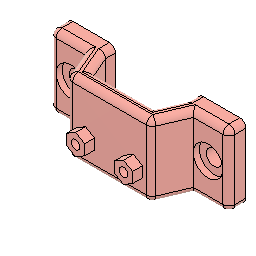
Z Leadscrew Nut to Bed Mount v7 (Autodesk Fusion 360 design; units mm, degrees)
Autodesk Fusion 360 part; units mm, degrees
sketch "Sketch1" plane through (0, 0, 0) normal (0, 0, 1) x (1, 0, 0) in component "Leadscrew Nut Mount V1"
  line L0 (0, 0) -> (0, 30)
  line L1 (0, 0) -> (73.8, 0)
  line L2 (73.8, 0) -> (73.8, 30)
  line L3 (73.8, 30) -> (0, 30)
  line L4 (36.9, 0) -> (36.9, 10) construction
  line L5 (36.9, 10) -> (27, 10) construction
  line L6 (36.9, 10) -> (46.8, 10) construction
  circle A0 centre (27, 10) radius 2.5
  circle A1 centre (46.8, 10) radius 2.5
  line L7 (29.9, 11.6743) -> (27, 13.3486)
  line L8 (27, 13.3486) -> (24.1, 11.6743)
  line L9 (24.1, 11.6743) -> (24.1, 8.3257)
  line L10 (24.1, 8.3257) -> (27, 6.6514)
  line L11 (27, 6.6514) -> (29.9, 8.3257)
  line L12 (29.9, 8.3257) -> (29.9, 11.6743)
  line L13 (43.9, 8.3257) -> (46.8, 6.6514)
  line L14 (46.8, 6.6514) -> (49.7, 8.3257)
  line L15 (49.7, 8.3257) -> (49.7, 11.6743)
  line L16 (49.7, 11.6743) -> (46.8, 13.3486)
  line L17 (46.8, 13.3486) -> (43.9, 11.6743)
  line L18 (43.9, 11.6743) -> (43.9, 8.3257)
  line L19 (0, 0) -> (20, 0)
  line L20 (20, 0) -> (20, 30)
  circle A2 centre (8.6, 15) radius 3.2
  circle A3 centre (8.6, 15) radius 6.1
  circle A4 centre (65.2, 15) radius 6.1
  circle A5 centre (65.2, 15) radius 3.2
  line L21 (53.8, 0) -> (53.8, 30)
  line L22 (0, 15) -> (8.6, 15) construction
  dimension "d1" = 10
  dimension "d2" = 5
  dimension "d3" = 5
  dimension "d4" = 9.9
  dimension "d5" = 2.9
  dimension "d6" = 2.9
  dimension "d21" = 73.8
  dimension "d22" = 6.4
  dimension "d23" = 12.2
  dimension "d24" = 30
  dimension "d25" = 33.8
  dimension "d26" = 8.6
  measures "d1" distance of L0.start
  measures "d2" diameter of A1
  measures "d3" diameter of A0
  measures "d5" distance of L18
  measures "d6" distance of L12
  measures "d22" diameter of A2
  measures "d23" diameter of A3
  measures "d25" distance of L20 L21
extrude "Extrude1" add sketch "Sketch1" along normal blind 7 contours L0 L1 L3 L19 L20 | L1 L2 L3 L21 | A3 | A4 makes body 1 at (64.187, 3.9363, 0) makes body 2 at (9.613, 3.9363, 0) in component "Leadscrew Nut Mount V1"
extrude "Extrude2" cut sketch "Sketch1" along normal through all from surface at 4.5 contours A3 | A4 bodies 1 2 in component "Leadscrew Nut Mount V1"
extrude "Extrude3" add sketch "Sketch1" along normal blind 2.75 from surface at 25.4 separate body contours L1 L3 L20 L21 makes body 3 in component "Leadscrew Nut Mount V1"
extrude "Extrude4" add sketch "Sketch1" along normal blind 3 from surface at 28.15 contours L1 L3 L20 L21 | L7 L8 L9 L10 L11 L12 | L13 L14 L15 L16 L17 L18 bodies 3 in component "Leadscrew Nut Mount V1"
sketch "Sketch2" plane through (0, 0, 0) normal (0, -1, 0) x (1, 0, 0) in component "Leadscrew Nut Mount V1"
  line L0 (20, 25.4) -> (53.8, 25.4)
  line L1 (53.8, 25.4) -> (53.8, 31.15)
  line L2 (53.8, 31.15) -> (20, 31.15)
  line L3 (20, 31.15) -> (20, 25.4)
  line L4 (59.1, 7) -> (71.3, 7)
  line L5 (53.8, 25.4) -> (53.8, 31.15)
  line L6 (53.8, 31.15) -> (59.1, 7)
  line L7 (53.8, 25.4) -> (48.2257, 25.4)
  line L8 (53.8, 0) -> (53.8, 7)
  line L9 (49.7, 25.4) -> (53.8, 6.7179)
  line L10 (59.1, 7) -> (53.8, 7)
  line L11 (53.8, 25.4) -> (20, 25.4)
  line L12 (20, 31.15) -> (53.8, 31.15)
  line L13 (36.9, 31.15) -> (36.9, 25.4)
  line L14 (24.1, 25.4) -> (20, 6.7179)
  line L15 (20, 31.15) -> (14.7, 7)
  line L16 (20, 25.4) -> (24.1, 25.4)
  line L17 (20, 25.4) -> (20, 31.15)
  line L18 (14.7, 7) -> (20, 7)
  line L19 (20, 0) -> (20, 7)
extrude "Extrude5" add sketch "Sketch2" against normal up to surface (30 mm away) contours L0 L3 L11 L14 L15 L16 L17 L18 L19 | L0 L1 L5 L6 L7 L8 L9 L10 L11 bodies 3 1 2 in component "Leadscrew Nut Mount V1"
fillet "Fillet1" radius 2.5 28 edges at (36.9, 30, 31.15) (17.35, 30, 19.075) (36.9, 30, 25.4) (22.05, 30, 16.059) (51.75, 30, 16.059) (56.45, 30, 19.075) (56.45, 0, 19.075) (51.75, 0, 16.059) (22.05, 0, 16.059) (17.35, 0, 19.075) (36.9, 0, 31.15) (53.8, 15, 31.15) (20, 15, 31.15) (20, 30, 3.359) (0, 30, 3.5) (7.35, 30, 7) (0, 15, 7) (7.35, 0, 7) (53.8, 30, 3.359) (66.45, 30, 7) (73.8, 30, 3.5) (73.8, 15, 7) (73.8, 0, 3.5) (66.45, 0, 7) (53.8, 0, 3.359) (36.9, 0, 25.4) (20, 0, 3.359) (0, 0, 3.5) on bodies 3 in component "Leadscrew Nut Mount V1"
sketch "Sketch1 (2)" plane through (0, 0, 0) normal (0, 0, 1) x (1, 0, 0) in component "Leadscrew Nut Mount V1.1"
  line L0 (0, 0) -> (0, 30)
  line L1 (0, 0) -> (73.8, 0)
  line L2 (73.8, 0) -> (73.8, 30)
  line L3 (73.8, 30) -> (0, 30)
  line L4 (36.9, 0) -> (36.9, 10) construction
  line L5 (36.9, 10) -> (27, 10) construction
  line L6 (36.9, 10) -> (46.8, 10) construction
  circle A0 centre (27, 10) radius 1.8
  circle A1 centre (46.8, 10) radius 1.8
  line L7 (29.9, 11.6743) -> (27, 13.3486)
  line L8 (27, 13.3486) -> (24.1, 11.6743)
  line L9 (24.1, 11.6743) -> (24.1, 8.3257)
  line L10 (24.1, 8.3257) -> (27, 6.6514)
  line L11 (27, 6.6514) -> (29.9, 8.3257)
  line L12 (29.9, 8.3257) -> (29.9, 11.6743)
  line L13 (43.9, 8.3257) -> (46.8, 6.6514)
  line L14 (46.8, 6.6514) -> (49.7, 8.3257)
  line L15 (49.7, 8.3257) -> (49.7, 11.6743)
  line L16 (49.7, 11.6743) -> (46.8, 13.3486)
  line L17 (46.8, 13.3486) -> (43.9, 11.6743)
  line L18 (43.9, 11.6743) -> (43.9, 8.3257)
  line L19 (0, 0) -> (20, 0)
  line L20 (20, 0) -> (20, 30)
  circle A2 centre (8.6, 15) radius 3.2
  circle A3 centre (8.6, 15) radius 6.1
  circle A4 centre (65.2, 15) radius 6.1
  circle A5 centre (65.2, 15) radius 3.2
  line L21 (53.8, 0) -> (53.8, 30)
  line L22 (0, 15) -> (8.6, 15) construction
  dimension "d1_1" = 10
  dimension "d2_1" = 3.6
  dimension "d3_1" = 3.6
  dimension "d4_1" = 9.9
  dimension "d5_1" = 2.9
  dimension "d6_1" = 2.9
  dimension "d21_1" = 73.8
  dimension "d22_1" = 6.4
  dimension "d23_1" = 12.2
  dimension "d24_1" = 30
  dimension "d25_1" = 33.8
  dimension "d26_1" = 8.6
  measures "d1_1" distance of L0.start
  measures "d2_1" diameter of A1
  measures "d3_1" diameter of A0
  measures "d5_1" distance of L18
  measures "d6_1" distance of L12
  measures "d22_1" diameter of A2
  measures "d23_1" diameter of A3
  measures "d25_1" distance of L20 L21
extrude "Extrude1'" add sketch "Sketch1 (2)" along normal blind 7 separate body contours L0 L1 L3 L19 L20 | L1 L2 L3 L21 | A3 | A4 makes body 4 at (64.187, 3.9363, 0) makes body 5 at (9.613, 3.9363, 0) in component "Leadscrew Nut Mount V1.1"
extrude "Extrude2'" cut sketch "Sketch1 (2)" along normal through all from surface at 4.5 contours A3 | A4 bodies 4 5 in component "Leadscrew Nut Mount V1.1"
extrude "Extrude3'" add sketch "Sketch1 (2)" along normal blind 2.75 from surface at 13.65 separate body contours L1 L3 L20 L21 makes body 6 in component "Leadscrew Nut Mount V1.1"
extrude "Extrude4'" add sketch "Sketch1 (2)" along normal blind 3 from surface at 16.4 contours L1 L3 L20 L21 | L7 L8 L9 L10 L11 L12 | L13 L14 L15 L16 L17 L18 bodies 6 in component "Leadscrew Nut Mount V1.1"
sketch "Sketch2 (2)" plane through (0, 0, 0) normal (0, -1, 0) x (1, 0, 0) in component "Leadscrew Nut Mount V1.1"
  line L0 (20, 13.65) -> (53.8, 13.65)
  line L1 (53.8, 13.65) -> (53.8, 19.4)
  line L2 (53.8, 19.4) -> (20, 19.4)
  line L3 (20, 19.4) -> (20, 13.65)
  line L4 (59.1, 7) -> (71.3, 7)
  line L5 (53.8, 13.65) -> (53.8, 19.4)
  line L6 (53.8, 19.4) -> (59.1, 7)
  line L7 (53.8, 13.65) -> (48.2257, 13.65)
  line L8 (53.8, 0) -> (53.8, 7)
  line L9 (49.7, 13.65) -> (53.8, 4.0575)
  line L10 (59.1, 7) -> (53.8, 7)
  line L11 (53.8, 13.65) -> (20, 13.65)
  line L12 (20, 19.4) -> (53.8, 19.4)
  line L13 (36.9, 19.4) -> (36.9, 13.65)
  line L14 (24.1, 13.65) -> (20, 4.0575)
  line L15 (20, 19.4) -> (14.7, 7)
  line L16 (20, 13.65) -> (24.1, 13.65)
  line L17 (20, 13.65) -> (20, 19.4)
  line L18 (14.7, 7) -> (20, 7)
  line L19 (20, 0) -> (20, 7)
extrude "Extrude5'" add sketch "Sketch2 (2)" against normal up to surface (30 mm away) contours L0 L3 L11 L14 L15 L16 L17 L18 L19 | L0 L1 L5 L6 L7 L8 L9 L10 L11 bodies 6 4 5 in component "Leadscrew Nut Mount V1.1"
fillet "Fillet1'" radius 2.5 28 edges at (36.9, 30, 19.4) (17.35, 30, 13.2) (36.9, 30, 13.65) (22.05, 30, 8.8538) (51.75, 30, 8.8538) (56.45, 30, 13.2) (56.45, 0, 13.2) (51.75, 0, 8.8538) (22.05, 0, 8.8538) (17.35, 0, 13.2) (36.9, 0, 19.4) (53.8, 15, 19.4) (20, 15, 19.4) (20, 30, 2.0288) (0, 30, 3.5) (7.35, 30, 7) (0, 15, 7) (7.35, 0, 7) (53.8, 30, 2.0288) (66.45, 30, 7) (73.8, 30, 3.5) (73.8, 15, 7) (73.8, 0, 3.5) (66.45, 0, 7) (53.8, 0, 2.0288) (36.9, 0, 13.65) (20, 0, 2.0288) (0, 0, 3.5) on bodies 6 in component "Leadscrew Nut Mount V1.1"
sketch "Sketch1 (1)" plane through (0, 0, 19.4) normal (0, 0, 1) x (1, 0, 0) in component "Leadscrew Nut Mount V1.1"
  circle A0 centre (46.8, 10) radius 1.8
  circle A1 centre (27, 10) radius 1.8
  line L0 (52.1498, 27.5) -> (21.6502, 27.5)
  line L1 (21.6502, 27.5) -> (21.6502, 2.5)
  line L2 (21.6502, 2.5) -> (52.1498, 2.5)
  line L3 (52.1498, 2.5) -> (52.1498, 27.5)
  line L4 (30.75, 12.1651) -> (27, 14.3301)
  line L5 (27, 14.3301) -> (23.25, 12.1651)
  line L6 (23.25, 12.1651) -> (23.25, 7.8349)
  line L7 (23.25, 7.8349) -> (27, 5.6699)
  line L8 (27, 5.6699) -> (30.75, 7.8349)
  line L9 (30.75, 7.8349) -> (30.75, 12.1651)
  line L10 (43.05, 7.8349) -> (46.8, 5.6699)
  line L11 (46.8, 5.6699) -> (50.55, 7.8349)
  line L12 (50.55, 7.8349) -> (50.55, 12.1651)
  line L13 (50.55, 12.1651) -> (46.8, 14.3301)
  line L14 (46.8, 14.3301) -> (43.05, 12.1651)
  line L15 (43.05, 12.1651) -> (43.05, 7.8349)
  dimension "d28" = 3.75
  dimension "d29" = 3.75
  measures "d28" distance of L9
  measures "d29" distance of L15
extrude "Extrude1''" add sketch "Sketch1 (1)" along normal blind 4.1 contours L4 L5 L6 L7 L8 L9 | L10 L11 L12 L13 L14 L15 bodies 6 in component "Leadscrew Nut Mount V1.1"
component "Leadscrew Nut Mount V1" placed x (1, 0, 0) y (0, 1, 0) z (0, 0, 1) at (0, 0, 0)
component "Leadscrew Nut Mount V1.1" placed x (1, 0, 0) y (0, 1, 0) z (0, 0, 1) at (0, 0, 0)
equation "d1 = d2 / 2 + 7.5 mm"
equation "d3 = d2"
equation "d4 = d2 / 2 + ( 14.8 / 2 ) * 1 mm"
equation "d6 = d5"
equation "d26 = d23 / 2 + 2.5 mm"
equation "d1_1 = ( 5 / 2 ) * 1 mm + 7.5 mm"
equation "d3_1 = d2_1"
equation "d4_1 = ( 5 / 2 ) * 1 mm + ( 14.8 / 2 ) * 1 mm"
equation "d6_1 = d5_1"
equation "d13_1 = 25.4 mm - 2.75 mm - 3 mm - 6 mm"
equation "d26_1 = d23_1 / 2 + 2.5 mm"
equation "d28 = d29"
equation "d29 = ( 7.9 / 2 ) * 1 mm - 0.2 mm"
